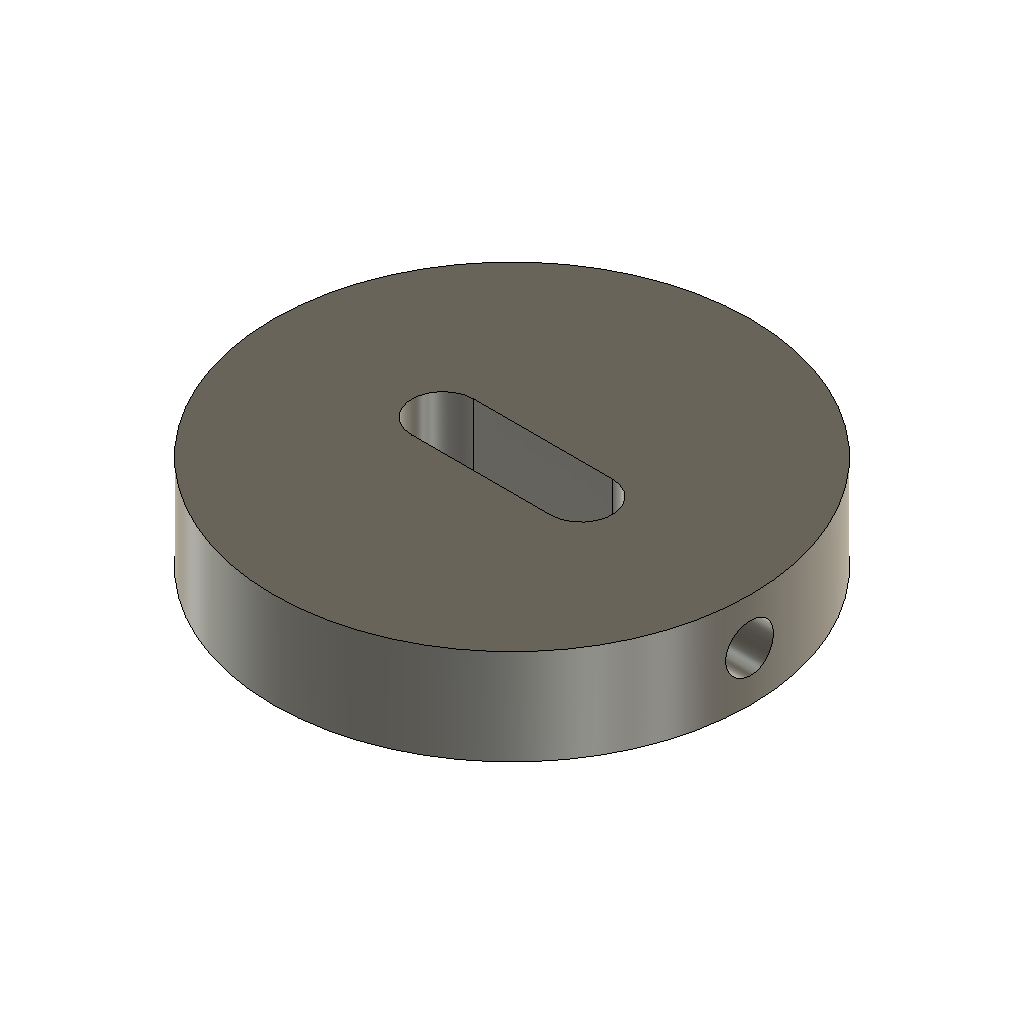
backplate (Autodesk Fusion 360 design; units mm, degrees)
part number: 2026-09-10-22-58-11-681
Autodesk Fusion 360 part; units mm, degrees
sketch "Sketch1" plane through (0, 0, 0) normal (0, 0, 1) x (1, 0, 0)
  circle A0 centre (0, 0) radius 10
  dimension "d1" = 20
  constraint coincident A0.centre origin
  measures "d1" diameter of A0
extrude "Extrude1" add sketch "Sketch1" along normal blind 3
sketch "Sketch2" plane through (0, 0, 3) normal (0, 0, 1) x (-1, 0, 0)
  circle A0 centre (0, 0) radius 10
  line L0 (-4.2, 1.3) -> (4.2, 1.3)
  line L1 (4.2, 1.3) -> (4.2, -1.3)
  line L2 (4.2, -1.3) -> (-4.2, -1.3)
  line L3 (-4.2, -1.3) -> (-4.2, 1.3)
  line L4 (-4.2, 1.3) -> (4.2, -1.3) construction
  line L5 (4.2, 1.3) -> (-4.2, -1.3) construction
  dimension "d4" = 8.4
  dimension "d5" = 2.6
  constraint horizontal L0
  constraint perpendicular L0 L1
  constraint parallel L0 L2
  constraint parallel L1 L3
  constraint coincident L4 A0.centre
  constraint coincident L5 A0.centre
  constraint coincident A0.centre origin
  measures "d4" distance of L1.end L2.end
  measures "d5" distance of L0.end L1.end
extrude "Extrude2" cut sketch "Sketch2" against normal blind 6 contours L0 L1 L2 L3
fillet "Fillet1" radius 1.3 4 edges at (4.2, 1.3, 1.5) (4.2, -1.3, 1.5) (-4.2, 1.3, 1.5) (-4.2, -1.3, 1.5)
extrude "Extrude3" add 1 faces at (-0.2491, -4.1907, 3) along direction (0, 0, 1) blind 1
hole "Hole1" at (10, 0, 2.0667) direction (-1, 0, 0) diameter 2 depth 4 tip angle 180
mirror "Mirror1" about plane through (0, 0, 0) normal (1, 0, 0) of "Hole1"
